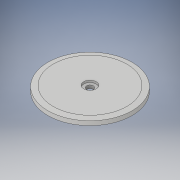
# Autodesk Inventor part: support_serrage_tourelle
Saved by Autodesk Inventor 2019 (Build 230136000, 136)
## iProperties
Created: 2018-05-17
Part Number: support_serrage_tourelle
Material: Générique
Document SubType Name: Modeling
Designer: Theo
Density: 1 g/cm^3
Appearance: Par défaut
Author: Theo
Autodesk Inventor part; units mm, degrees
ref_plane "YZ Plane" through (0, 0, 0) normal (1, 0, 0) x (0, 1, 0)
ref_plane "XZ Plane" through (0, 0, 0) normal (0, 1, 0) x (-1, 0, 0)
ref_plane "XY Plane" through (0, 0, 0) normal (0, 0, 1) x (1, 0, 0)
sketch "Esquisse3" plane through (0, 0, 0) normal (1, 0, 0) x (0, 1, 0)
  line L0 (-7.2956, 0) -> (7.2956, 0)
  line L1 (5, 0) -> (5, 35)
  line L2 (5, 35) -> (4, 40)
  line L3 (4, 40) -> (0, 40)
  line L4 (0, 40) -> (0, 0)
  line L5 (0, 0) -> (5, 0)
  dimension "d1" = 5
  dimension "d2" = 4
  dimension "d3" = 5
  dimension "d4" = 80
  constraints: 12 end point, 3 horizontal, 2 vertical, 1 coincident, 1 midpoint
  measures "d1" distance between parallel lines of L1 L4
  measures "d2" distance of L3.end L2.end
  measures "d3" vertical distance of L1.end L2.end
  measures "d4" diameter of L3 L0
revolve "Révolution1" add sketch "Esquisse3" angle 360 about axis through (0, -7.2956, 0) along (0, 1, 0)
sketch "Esquisse4" plane through (0, 5, 0) normal (0, 1, 0) x (1, 0, 0)
  point P0 (0, 0)
  point P1 (0, 0)
  constraints: 1 coincident
hole "Perçage1" at (0, 5, 0) direction (0, -1, 0) diameter 6.4 end through all counterbore diameter 12 counterbore depth 2
sketch "Esquisse5" plane through (0, 0, 0) normal (0, -1, 0) x (1, 0, 0)
  circle A0 centre (0, 30) radius 2
  point P0 (0, 0)
  dimension "d13" = 4
  dimension "d14" = 30
  constraints: 1 centre point, 1 vertical alignment
  measures "d13" diameter of A0
  measures "d14" distance of point (0, 0) A0.centre
extrude "Extrusion1" add sketch "Esquisse5" along normal blind 2.8
chamfer "Chanfrein1" distance 1.5 angle 45 1 edges at (-2, -2.8, 30)
pattern_circular "Réseau circulaire1" count 3 over 360 about axis through (0, -10, 0) along (0, 1, 0) of "Extrusion1", "Chanfrein1"
